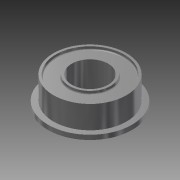
# Autodesk Inventor part: 40
Saved by Autodesk Inventor 2013 (Build 170138000, 138)
## iProperties
Created: 2013-04-08
Material: ステンレス鋼
Document SubType Name: Modeling
Designer: andou
Density: 8.08 g/cm^3
Description: MF84ZZ
Mass: 0.843551 g
Surface Area: 2.42185 cm^2
Volume: 0.1044 cm^3
Part Number: 40
Author: andou
Title: Bearing
Autodesk Inventor part; units mm, degrees
ref_plane "YZ Plane" through (0, 0, 0) normal (1, 0, 0) x (0, 1, 0)
ref_plane "XZ Plane" through (0, 0, 0) normal (0, 1, 0) x (-1, 0, 0)
ref_plane "XY Plane" through (0, 0, 0) normal (0, 0, 1) x (1, 0, 0)
sketch "スケッチ1" plane through (0, 0, 0) normal (0, 0, 1) x (1, 0, 0)
  circle A0 centre (0, 0) radius 4.6
  dimension "d0" = 9.2
  constraints: 1 centre point, 1 coincident
  measures "d0" diameter of A0
extrude "押し出し1" add sketch "スケッチ1" along normal blind 0.5
sketch "スケッチ2" plane through (0, 0, 0.5) normal (0, 0, 1) x (1, 0, 0)
  circle A0 centre (0, 0) radius 4.6 projected
  circle A1 centre (0, 0) radius 4
  dimension "d3" = 8
  constraints: 1 centre point, 1 coincident
  measures "d3" diameter of A1
extrude "押し出し2" add sketch "スケッチ2" along normal blind 2.5 contours A1
sketch "スケッチ3" plane through (0, 0, 3) normal (0, 0, 1) x (1, 0, 0)
  circle A0 centre (0, 0) radius 4 projected
  circle A1 centre (0, 0) radius 2
  dimension "d6" = 4
  constraints: 1 centre point, 1 coincident
  measures "d6" diameter of A1
hole "穴1" at (0, 0, 3) direction (0, 0, -1) diameter 4 end through all
sketch "スケッチ4" plane through (0, 0, 3) normal (0, 0, 1) x (1, 0, 0)
  circle A0 centre (0, 0) radius 4 projected
  circle A1 centre (0, 0) radius 3.75
  circle A2 centre (0, 0) radius 2.25
  dimension "d14" = 4.5
  dimension "d15" = 7.5
  constraints: 2 centre point, 2 coincident
  measures "d14" diameter of A2
  measures "d15" diameter of A1
extrude "押し出し3" cut sketch "スケッチ4" against normal blind 0.3 contours A1
sketch "スケッチ5" plane through (0, 0, 0) normal (0, 0, -1) x (-1, 0, 0)
  circle A0 centre (0, 0) radius 4.6 projected
  circle A1 centre (0, 0) radius 3.75
  circle A2 centre (0, 0) radius 2.25
  dimension "d18" = 4.5
  dimension "d19" = 7.5
  constraints: 2 centre point, 2 coincident
  measures "d18" diameter of A2
  measures "d19" diameter of A1
extrude "押し出し4" cut sketch "スケッチ5" against normal blind 0.3 contours A1
fillet "フィレット1" radius 0.1 4 edges at (2.25, 0, 0.3) (3.75, 0, 0.3) (-2.25, 0, 2.7) (-3.75, 0, 2.7)
